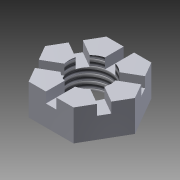
# Autodesk Inventor part: 砂轮架固定销螺丝
Saved by Autodesk Inventor 2015 (Build 190159000, 159)
## iProperties
Created: 2017-05-17
Part Number: 砂轮架固定销螺丝
Material: 常规
Document SubType Name: Modeling
Designer: Administrator
Density: 1 g/cm^3
Appearance: PTFE
Author: Administrator
Autodesk Inventor part; units mm, degrees
ref_plane "YZ Plane" through (0, 0, 0) normal (1, 0, 0) x (0, 1, 0)
ref_plane "XZ Plane" through (0, 0, 0) normal (0, 1, 0) x (-1, 0, 0)
ref_plane "XY Plane" through (0, 0, 0) normal (0, 0, 1) x (1, 0, 0)
sketch "草图2" plane through (0, 0, 0) normal (0, 0, 1) x (1, 0, 0)
  line L0 (4.3301, -7.5) -> (-4.3301, -7.5)
  line L1 (-4.3301, -7.5) -> (-8.6603, 0)
  line L2 (-8.6603, 0) -> (-4.3301, 7.5)
  line L3 (-4.3301, 7.5) -> (4.3301, 7.5)
  line L4 (4.3301, 7.5) -> (8.6603, 0)
  line L5 (8.6603, 0) -> (4.3301, -7.5)
  line L6 (0, 0) -> (0, 3.4444)
  circle A0 centre (0, 0) radius 4
  point P0 (0, 7.5)
  dimension "d6" = 3.4444
  dimension "d7" = 15
  dimension "d8" = 8
  constraints: 14 end point, 3 coincident, 1 centre point, 1 midpoint, 1 point on line, 1 vertical, 13 other
  measures "d6" distance of L6.start L6.end
  measures "d7" distance between parallel lines of L0 L3
  measures "d8" diameter of A0
extrude "拉伸2" add sketch "草图2" along normal blind 6
thread "螺纹1" size "M8x1.25" class "6H" standard "ANSI Metric M Profile" full length
sketch "草图3" plane through (0, 0, 6) normal (0, 0, 1) x (1, 0, 0)
  line L0 (-4.3301, -7.5) -> (4.3301, -7.5) projected
  line L1 (-1, 7.5) -> (1, 7.5)
  line L2 (1, 7.5) -> (1, -7.5)
  line L3 (1, -7.5) -> (-1, -7.5)
  line L4 (-1, -7.5) -> (-1, 7.5)
  point P0 (0, 0)
  dimension "d13" = 2
  dimension "d14" = 1
  dimension "d15" = 15
  constraints: 8 end point, 2 parallel, 1 horizontal, 1 perpendicular, 1 point on line
  measures "d13" distance of L1.start L1.end
  measures "d14" distance from line of L2 point (0, 0)
  measures "d15" distance of L1.end L2.end
extrude "拉伸3" cut sketch "草图3" against normal blind 2
pattern_circular "环形阵列1" count 3 over 360 about axis through (0, 0, -10) along (0, 0, 1) of "拉伸3"
